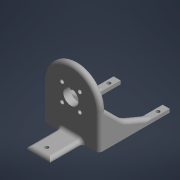
# Autodesk Inventor part: 5202 Series Yellow Jacket planetary Gear Motor Mount
Saved by Autodesk Inventor 2022 (Build 260153000, 153)
## iProperties
Part Number: 5202 Series Yellow Jacket planetary Gear Motor Mount
Material: Generic
Document SubType Name: Modeling
Designer: izack
Appearance: Default
Author: izack
Autodesk Inventor part; units mm, degrees
ref_plane "YZ Plane" through (0, 0, 0) normal (1, 0, 0) x (0, 1, 0)
ref_plane "XZ Plane" through (0, 0, 0) normal (0, 1, 0) x (-1, 0, 0)
ref_plane "XY Plane" through (0, 0, 0) normal (0, 0, 1) x (1, 0, 0)
sketch "Sketch1" plane through (0, 0, 0) normal (0, 1, 0) x (-1, 0, 0)
  line L0 (0, 0) -> (50.8, 0)
  line L1 (50.8, 0) -> (50.8, -93.4974)
  line L2 (50.8, -93.4974) -> (0, -93.4974)
  line L3 (0, -93.4974) -> (0, 0)
  dimension "d0" = 50.8
  dimension "d1" = 93.4974
  constraints: 8 end point, 2 parallel, 1 horizontal, 1 perpendicular
  measures "d0" distance of L1.end L2.end
  measures "d1" distance of L0.end L1.end
extrude "Extrusion1" add sketch "Sketch1" along normal blind 3.0988
sketch "Sketch2" plane through (0, 3.0988, 0) normal (0, 1, 0) x (1, 0, 0)
  circle A0 centre (-25.4, 7.5) radius 1.7
  line L0 (0, 0) -> (0, 93.4974) projected
  line L1 (-50.8, 0) -> (0, 0) projected
  line L2 (-50.8, 93.4974) -> (-50.8, 0) projected
  line L3 (-50.8, 29.5) -> (0, 29.5)
  line L4 (-35.8, 29.5) -> (-35.8, 0)
  line L5 (-25.4, 0) -> (-25.4, 93.4974)
  line L6 (0, 93.4974) -> (-50.8, 93.4974) projected
  line L7 (-50.8, 35.85) -> (0, 35.85)
  line L8 (-44.45, 35.85) -> (-44.45, 93.4974)
  line L9 (-6.35, 35.85) -> (-6.35, 93.4974)
  line L10 (-15, 29.5) -> (-15, 0)
  circle A1 centre (-47.625, 85.9974) radius 1.7
  circle A2 centre (-3.175, 85.9974) radius 1.7
  line L11 (-50.8, 92.4833) -> (-44.45, 92.4833)
  line L12 (-47.625, 92.4833) -> (-47.625, 77.1413)
  line L13 (-6.35, 91.9271) -> (0, 91.9271)
  line L14 (-3.175, 91.9271) -> (-3.175, 75.8899)
  dimension "d4" = 3.4
  dimension "d5" = 25.4
  dimension "d6" = 7.5
  dimension "d7" = 22
  dimension "d8" = 6.35
  dimension "d10" = 15
  dimension "d11" = 15
  dimension "d12" = 6.35
  dimension "d13" = 6.35
  dimension "d14" = 3.4
  dimension "d15" = 3.4
  dimension "d16" = 7.5
  dimension "d17" = 7.5
  constraints: 22 end point, 18 point on line, 7 perpendicular, 4 midpoint, 3 centre point, 2 vertical, 1 horizontal
  measures "d4" diameter of A0
  measures "d5" distance from line of L0 A0.centre
  measures "d6" distance from line of L1 A0.centre
  measures "d7" distance from line of L3 A0.centre
  measures "d8" distance between parallel lines of L7 L3
  measures "d10" distance between parallel lines of L2 L4
  measures "d11" distance between parallel lines of L0 L10
  measures "d12" distance between parallel lines of L8 L2
  measures "d13" distance between parallel lines of L0 L9
  measures "d14" diameter of A2
  measures "d15" diameter of A1
  measures "d16" distance from line of L6 A2.centre
  measures "d17" distance from line of L6 A1.centre
extrude "Extrusion2" cut sketch "Sketch2" against normal blind 3.0988 contours A0 L5 | L5 A0 | L4 L1 L2 L3 | L3 L0 L1 L10 | L7 L8 L6 L5 | L5 L6 L9 L7 | A1 L12 | L12 A1 | A2 L14 | L14 A2
sketch "Sketch3" plane through (0, 3.0988, 0) normal (0, 1, 0) x (1, 0, 0)
  line L0 (-35.8, 0) -> (-35.8, 29.5) projected
  line L1 (0, 29.5) -> (-15, 29.5) projected
  line L2 (-35.8, 29.5) -> (-15, 29.5)
  circle A0 centre (-3.175, 85.9974) radius 1.7 projected
  circle A1 centre (-47.625, 85.9974) radius 1.7 projected
  line L3 (-50.8, 93.4974) -> (-50.8, 29.5) projected
  line L4 (-50.8, 29.5) -> (-35.8, 29.5) projected
  line L5 (-6.35, 35.85) -> (-44.45, 35.85) projected
  line L6 (-44.45, 35.85) -> (-44.45, 93.4974) projected
  line L7 (-15, 29.5) -> (0, 29.5) projected
  line L8 (0, 29.5) -> (0, 93.4974) projected
  line L9 (0, 93.4974) -> (-6.35, 93.4974) projected
  line L10 (-6.35, 93.4974) -> (-6.35, 35.85) projected
  line L11 (-6.35, 35.85) -> (-44.45, 35.85) projected
  line L12 (-44.45, 35.85) -> (-44.45, 93.4974) projected
  line L13 (-44.45, 93.4974) -> (-50.8, 93.4974) projected
  line L14 (-50.8, 93.4974) -> (-50.8, 29.5) projected
  line L15 (-50.8, 29.5) -> (-35.8, 29.5) projected
  line L16 (-35.8, 29.5) -> (-35.8, 0) projected
  line L17 (-35.8, 0) -> (-15, 0) projected
  line L18 (-15, 0) -> (-15, 29.5) projected
  circle A2 centre (-47.625, 85.9974) radius 1.7 projected
  circle A3 centre (-25.4, 7.5) radius 1.7 projected
  circle A4 centre (-3.175, 85.9974) radius 1.7 projected
  line L19 (-44.45, 35.85) -> (-50.8, 35.85)
  line L20 (-6.35, 93.4974) -> (-6.35, 35.85) projected
  line L21 (-6.35, 35.85) -> (0, 35.85)
  line L22 (0, 29.5) -> (0, 93.4974) projected
  point P0 (0, 0)
  point P1 (0, 35.85)
  constraints: 6 end point, 3 point on line, 1 horizontal, 1 perpendicular
extrude "Extrusion3" add sketch "Sketch3" along normal blind 53.848 contours L4 L3 L19 L5 L21 L8 L1 L2
fillet "Fillet1" radius 25.35 2 edges at (0, 56.9468, -32.675) (-50.8, 56.9468, -32.675)
chamfer "Chamfer1" distance 27.5 angle 45 2 edges at (-3.175, 3.0988, -35.85) (-47.625, 3.0988, -35.85)
chamfer "Chamfer2" distance 15.25 angle 45 2 edges at (-3.175, 3.0988, -63.35) (-47.625, 3.0988, -63.35)
fillet "Fillet2" radius 25.35 2 edges at (-3.175, 13.8822, -52.5666) (-47.625, 13.8822, -52.5666)
fillet "Fillet3" radius 3.1 3 edges at (-15, 3.0988, -14.75) (-25.4, 3.0988, 0) (-35.8, 3.0988, -14.75)
fillet "Fillet4" radius 3.1 22 edges at (-25.4, 56.9468, -35.85) (-43.3752, 49.522, -35.85) (-50.8, 31.0978, -35.85) (0, 31.0978, -35.85) (-7.4248, 49.522, -35.85) (0, 15.7984, -29.5) (-25.4, 56.9468, -29.5) (-43.3752, 49.522, -29.5) (-50.8, 15.7984, -29.5) (-7.4248, 49.522, -29.5) (0, 14.2951, -52.8425) (0, 7.5257, -67.9126) (0, 24.0233, -42.4255) (-6.35, 14.2951, -52.8425) (-6.35, 7.5257, -67.9126) (-6.35, 24.0233, -42.4255) (-50.8, 14.2951, -52.8425) (-50.8, 7.5257, -67.9126) (-50.8, 24.0233, -42.4255) (-44.45, 14.2951, -52.8425) (-44.45, 7.5257, -67.9126) (-44.45, 24.0233, -42.4255)
sketch "Sketch4" plane through (-32.7, 3.0988, -29.5) normal (0, 0, 1) x (1, 0, 0)
  arc A0 (7.25, 53.848) -> (-18.1, 28.498) centre (7.25, 28.498) ccw projected
  line L0 (5.6, 0) -> (9, 0) projected
  line L1 (-18.1, 26.2159) -> (-18.1, 28.498) projected
  line L2 (32.7, 28.498) -> (29.6, 28.498) projected
  circle A1 centre (-0.75, 36.498) radius 1.7
  circle A2 centre (-0.75, 20.498) radius 1.7
  circle A3 centre (15.25, 36.498) radius 1.7
  circle A4 centre (15.25, 20.498) radius 1.7
  circle A5 centre (7.25, 28.498) radius 6.862
  line L3 (7.25, 53.848) -> (7.25, 0)
  line L4 (7.25, 53.848) -> (61.098, 53.848) construction
  line L5 (7.25, 28.498) -> (-18.1, 28.498)
  line L6 (-0.75, 20.498) -> (15.25, 20.498)
  line L7 (15.25, 20.498) -> (15.25, 36.498)
  line L8 (15.25, 36.498) -> (-0.75, 36.498)
  line L9 (-0.75, 36.498) -> (-0.75, 20.498)
  line L10 (-0.75, 20.498) -> (15.25, 36.498) construction
  line L11 (15.25, 20.498) -> (-0.75, 36.498) construction
  point P0 (32.7, -3.0988)
  dimension "d40" = 3.4
  dimension "d43" = 13.724
  dimension "d45" = 90
  dimension "d46" = 16
  dimension "d47" = 16
  constraints: 18 end point, 5 centre point, 5 coincident, 3 horizontal, 2 midpoint, 2 parallel, 2 perpendicular, 1 point on line
  measures "d40" diameter of A1
  measures "d43" diameter of A5
  measures "d45" angle of L3 L4
  measures "d46" distance of L8.end L7.end
  measures "d47" distance of L7.end L6.end
extrude "Extrusion4" cut sketch "Sketch4" against normal blind 13.724 contours L3 L5 A5 | A5 L3 | L8 L7 A3 | A3 L7 L8 | L8 L9 A1 | A1 L9 L8 | L5 L3 A5 | L9 L6 A2 | A2 L6 L9 | L7 L6 A4 | A4 L6 L7
fillet "Fillet5" radius 3.1 5 edges at (-35.8, 0.0009, -29.5) (-34.8929, 2.1917, -29.5) (-15.9071, 2.1917, -29.5) (-15, 0.0009, -29.5) (-25.4, 3.0988, -29.5)
equation "\"d38\" = d43"
body "Solid1"
